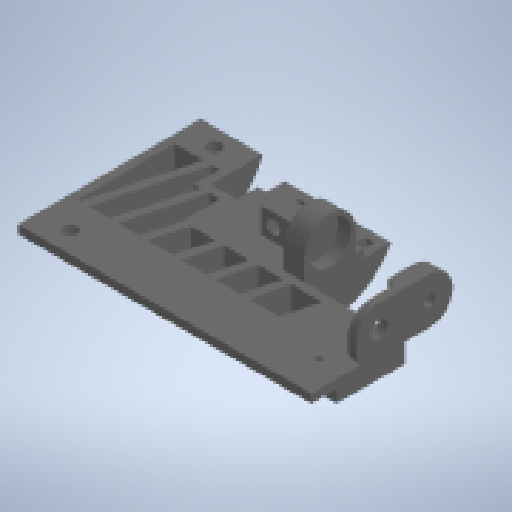
# Autodesk Inventor part: hand_motor_setter_cover_under
Saved by Autodesk Inventor 2024.1 (Build 281209000, 209)
## iProperties
Created: 2025-01-23
Part Number: hand_motor_setter_cover_under
Material: 一般
Document SubType Name: Modeling
Designer: hibik
Density: 1 g/cm^3
Appearance: 既定
Author: hibik
Autodesk Inventor part; units mm, degrees
ref_plane "YZ Plane" through (0, 0, 0) normal (1, 0, 0) x (0, 1, 0)
ref_plane "XZ Plane" through (0, 0, 0) normal (0, 1, 0) x (-1, 0, 0)
sketch "スケッチ1" plane through (0, 0, 0) normal (0, 1, 0) x (-1, 0, 0)
  line L0 (0, 0) -> (-14.7, 0)
  line L1 (-14.7, 0) -> (-14.7, -44.2)
  line L2 (-14.7, -44.2) -> (0, -44.2)
  line L3 (0, -44.2) -> (0, 0)
  line L4 (-14.7, -36.2) -> (-69.7, -36.2)
  line L5 (-69.7, -36.2) -> (-69.7, -22.1)
  line L6 (-69.7, -22.1) -> (-14.7, -22.1)
  line L7 (-14.7, -22.1) -> (-14.7, -36.2)
  line L8 (-7.35, -44.2) -> (-7.35, 0) construction
  circle A0 centre (-7.35, -39.2) radius 1.6
  circle A1 centre (-7.35, -5) radius 1.6
  point P0 (-14.7, -22.1)
  dimension "d0" = 14.7
  dimension "d1" = 44.2
  dimension "d2" = 22.1
  dimension "d3" = 14.1
  dimension "d4" = 3.2
  dimension "d5" = 3.2
  dimension "d6" = 5
  dimension "d7" = 5
  dimension "d20" = 55
  constraints: 18 end point, 4 parallel, 3 point on line, 2 centre point, 2 horizontal, 2 midpoint, 2 perpendicular
  measures "d0" distance of L2.end L1.end
  measures "d1" distance of L1.end L0.end
  measures "d2" distance between parallel lines of L2 L6
  measures "d3" distance between parallel lines of L6 L4
  measures "d4" diameter of A0
  measures "d5" diameter of A1
  measures "d6" distance of L8.start A0.centre
  measures "d7" distance from line of L0 A1.centre
  measures "d20" distance of L4.start L4.end
extrude "押し出し1" add sketch "スケッチ1" along normal blind 2
ref_plane "作業平面1" through (31, 0, -44.2) normal (-1, 0, 0) x (0, 0, 1)
sketch "スケッチ3" plane through (31, 0, -44.2) normal (-1, 0, 0) x (0, 0, 1)
  line L0 (22.1, 0) -> (8, 0) projected
  line L1 (8, 0) -> (8, 2) projected
  line L2 (22.1, 2) -> (8, 2) projected
  line L3 (22.1, 0) -> (22.1, 2) projected
  line L4 (17.45, 2) -> (12.65, 2)
  line L5 (12.65, 2) -> (12.65, 8)
  line L6 (12.65, 8) -> (17.45, 8)
  line L7 (17.45, 8) -> (17.45, 2)
  line L8 (22.1, 0) -> (8, 0) projected
  point P0 (44.2, 0)
  point P1 (15.05, 8)
  point P2 (15.05, 0)
  point P3 (12.65, 2)
  dimension "d11" = 4.8
  dimension "d12" = 6
  constraints: 8 end point, 2 midpoint, 2 parallel, 1 horizontal, 1 perpendicular, 1 point on line, 1 vertical alignment
  measures "d11" distance of L5.end L6.end
  measures "d12" distance of L6.end L4.start
extrude "押し出し2" add sketch "スケッチ3" against normal blind 5.9 contours L2 L5 L6 L7
sketch "スケッチ4" plane through (31, 2, -26.75) normal (0, 0, 1) x (1, 0, 0)
  circle A0 centre (2.9, 3) radius 1.6
  line L0 (5.9, 6) -> (5.9, 0) projected
  line L1 (0, 6) -> (5.9, 6) projected
  point P0 (-31, -2)
  dimension "d15" = 3.2
  dimension "d16" = 3
  dimension "d17" = 3
  constraints: 1 centre point
  measures "d15" diameter of A0
  measures "d16" distance from line of L0 A0.centre
  measures "d17" distance from line of L1 A0.centre
extrude "押し出し3" cut sketch "スケッチ4" against normal through all
sketch "スケッチ5" plane through (69.7, 0, -22.1) normal (1, 0, 0) x (0, 0, -1)
  circle A0 centre (-6, 7.1) radius 2 projected
  line L0 (0, 0) -> (14.1, 0) projected
  line L1 (14.1, 0) -> (14.1, 2) projected
  line L2 (0, 2) -> (14.1, 2) projected
  line L3 (0, 0) -> (0, 2) projected
  line L4 (14.1, 0) -> (22.1, 0) projected
  line L5 (14.1, 0) -> (-11.5, 0)
  line L6 (-11.5, 0) -> (-11.5, 12.6)
  line L7 (-11.5, 12.6) -> (14.1, 12.6)
  line L8 (14.1, 12.6) -> (14.1, 0)
  circle A1 centre (-6, 7.1) radius 5.5
  circle A2 centre (-6, 5.5) radius 5.5
  point P0 (-22.1, 0)
  point P1 (-11.5, 7.1)
  point P2 (-6, 12.6)
  point P3 (-11.5, 5.5)
  point P4 (-6, 0)
  dimension "d21" = 5.5
  dimension "d22" = 5.5
  constraints: 8 end point, 3 tangent, 2 centre point, 2 parallel, 1 coincident, 1 equal radius, 1 horizontal, 1 perpendicular
  measures "d21" distance from line of L6 A0.centre
  measures "d22" distance from line of L7 A0.centre
extrude "押し出し4" add sketch "スケッチ5" against normal blind 2 contours L3 L2 L1 L0 | L5 A2 A1 L7 L8 L2 L3 | A2 A1 | L6 A1 A2 | A1 A2 | A2 A1
sketch "スケッチ6" plane through (0, 0, 0) normal (0, -1, 0) x (1, 0, 0)
  line L0 (14.7, 0) -> (69.7, 0)
  line L1 (69.7, 0) -> (69.7, -22.1)
  line L2 (69.7, -22.1) -> (14.7, -22.1)
  line L3 (14.7, -22.1) -> (14.7, 0)
  line L4 (14.7, -22.1) -> (67.7, -22.1) projected
  line L5 (69.7, -16.1) -> (69.7, -36.2) projected
  point P0 (0, 0)
  constraints: 8 end point, 2 parallel, 1 coincident, 1 collinear, 1 horizontal, 1 perpendicular, 1 point on line
extrude "押し出し5" add sketch "スケッチ6" against normal up to surface (2 mm away)
sketch "スケッチ7" plane through (31, 2, -31.55) normal (0, 0, -1) x (-1, 0, 0)
  line L0 (-5.9, 0) -> (-5.9, 6) projected
  line L1 (-5.9, 6) -> (-36.7, 6)
  line L2 (-36.7, 6) -> (-36.7, 0)
  line L3 (-36.7, 0) -> (-5.9, 0)
  line L4 (-5.9, 0) -> (-5.9, 6)
  line L5 (-36.7, 10.6) -> (-36.7, 0) projected
  line L6 (-36.7, 0) -> (16.3, 0) projected
  point P0 (31, -2)
  point P1 (-36.7, 3)
  point P2 (-33.7, 0)
  constraints: 8 end point, 2 collinear, 2 parallel, 1 horizontal, 1 perpendicular
extrude "押し出し6" add sketch "スケッチ7" against normal up to surface (4.8 mm away)
ref_plane "作業平面2" through (41, 0, -44.2) normal (-1, 0, 0) x (0, 0, 1)
sketch "スケッチ8" plane through (41, 0, -44.2) normal (-1, 0, 0) x (0, 0, 1)
  circle A0 centre (16.1, 7.1) radius 2
  circle A1 centre (16.1, 7.1) radius 6
  line L0 (0, 2) -> (44.2, 2) projected
  line L1 (22.1, 7.1) -> (22.1, 2)
  line L2 (10.1, 7.1) -> (10.1, 0.8912)
  point P0 (44.2, 0)
  point P1 (10.1, 2)
  dimension "d38" = 12
  constraints: 4 end point, 2 centre point, 2 perpendicular, 2 point on circle, 2 tangent, 1 coincident, 1 midpoint, 2 other
  measures "d38" diameter of A1
extrude "押し出し7" add sketch "スケッチ8" against normal blind 5 contours A0 | A1 L0 | L1 L0 A1 | A1 L0 L2 picked at (16.1804, 3.0382)
sketch "スケッチ9" plane through (46, 0, -44.2) normal (1, 0, 0) x (0, 0, -1)
  line L0 (-12.65, 8) -> (-17.45, 8) projected
  line L1 (-12.65, 2) -> (-12.65, 8) projected
  line L2 (-17.45, 8) -> (-17.45, 2) projected
  line L3 (-12.55, 2) -> (-17.55, 2)
  point P0 (-44.2, 0)
  constraints: 2 end point, 1 horizontal, 2 other
extrude "押し出し8" cut sketch "スケッチ9" along normal blind 15
sketch "スケッチ10" plane through (0, 2, 0) normal (0, 1, 0) x (1, 0, 0)
  line L0 (46, 22.1) -> (46, 34.1) projected
  line L1 (46, 22.1) -> (61, 22.1)
  line L2 (61, 22.1) -> (61, 36.2)
  line L3 (61, 36.2) -> (46, 36.2)
  line L4 (46, 36.2) -> (46, 22.1)
  line L5 (61, 31.55) -> (61, 26.75) projected
  line L6 (67.7, 36.2) -> (14.7, 36.2) projected
  line L7 (19.8, 34.2) -> (14.8, 34.2)
  line L8 (14.7, 36.2) -> (19.8, 36.2)
  line L9 (19.8, 36.2) -> (19.8, 34.2)
  line L10 (19.8, 34.2) -> (14.7, 34.2)
  line L11 (14.7, 34.2) -> (14.7, 36.2)
  line L12 (19.8, 34.2) -> (20.8, 34.2)
  line L13 (20.8, 34.2) -> (20.8, 36.2)
  line L14 (20.8, 36.2) -> (19.8, 36.2)
  line L15 (19.8, 36.2) -> (19.8, 34.2)
  point P0 (0, 0)
  point P1 (64.7, 36.2)
  dimension "d37" = 1
  constraints: 26 end point, 6 parallel, 4 horizontal, 3 perpendicular, 2 collinear, 1 point on line, 2 other
  measures "d37" distance between parallel lines of L9 L13
extrude "押し出し9" cut sketch "スケッチ10" against normal through all
sketch "スケッチ11" plane through (46, 0, -44.2) normal (1, 0, 0) x (0, 0, -1)
  arc A0 (-10.1, 7.1) -> (-22.1, 7.1) centre (-16.1, 7.1) ccw projected
  circle A1 centre (-16.1, 7.1) radius 5
  point P0 (-44.2, 0)
  dimension "d39" = 10
  constraints: 1 centre point, 1 coincident
  measures "d39" diameter of A1
extrude "押し出し10" cut sketch "スケッチ11" against normal blind 3
sketch "スケッチ12" plane through (67.7, 0, -22.1) normal (-1, 0, 0) x (0, 0, 1)
  line L0 (0, 2) -> (0, 7.1) projected
  line L1 (6, 12.6) -> (-14.1, 12.6) projected
  line L2 (0, 2) -> (-14.1, 2)
  line L3 (-14.1, 2) -> (-14.1, 12.6)
  line L4 (-14.1, 12.6) -> (0, 12.6)
  line L5 (0, 12.6) -> (0, 2)
  point P0 (22.1, 0)
  point P1 (0, 7.1)
  constraints: 8 end point, 2 parallel, 1 horizontal, 1 perpendicular
extrude "押し出し11" add sketch "スケッチ12" along normal blind 3
fillet "フィレット3" radius 2.5 6 edges at (64.7, 2, -24.425) (62.85, 2, -26.75) (62.85, 8, -26.75) (62.85, 8, -31.55) (62.85, 2, -31.55) (64.7, 2, -33.875)
sketch "スケッチ13" plane through (61, 0, -44.2) normal (-1, 0, 0) x (0, 0, 1)
  circle A0 centre (15.05, 5.504) radius 1.6
  circle A1 centre (15.05, 5.504) radius 1.35
  point P0 (44.2, 0)
  dimension "d46" = 2.7
  constraints: 2 centre point, 1 coincident, 2 other
  measures "d46" diameter of A1
extrude "押し出し12" cut sketch "スケッチ13" against normal through all contours A1
sketch "スケッチ14" plane through (0, 0, 0) normal (0, -1, 0) x (1, 0, 0)
  circle A0 centre (63.3, -17.5) radius 1.25
  line L0 (69.7, 0) -> (69.7, -36.2) projected
  line L1 (54.7, -22.1) -> (69.7, -22.1)
  line L2 (69.7, -22.1) -> (69.7, -6)
  line L3 (69.7, -6) -> (54.7, -6)
  line L4 (54.7, -6) -> (54.7, -22.1)
  line L5 (46, -22.1) -> (61, -22.1) projected
  circle A1 centre (63.3, -8) radius 1.25
  circle A2 centre (63.3, -8) radius 0.85
  circle A3 centre (63.3, -17.5) radius 0.85
  point P0 (0, 0)
  dimension "d49" = 15
  dimension "d50" = 2
  dimension "d53" = 1.7
  dimension "d54" = 1.7
  constraints: 8 end point, 4 centre point, 2 coincident, 2 parallel, 1 collinear, 1 horizontal, 1 perpendicular, 1 point on line, 4 other
  measures "d49" distance of L1.start L1.end
  measures "d50" distance from line of L3 A1.centre
  measures "d53" diameter of A2
  measures "d54" diameter of A3
extrude "押し出し13" add sketch "スケッチ14" along normal blind 3 contours A0 | L0 L1 L4 L3 | A1
sketch "スケッチ15" plane through (0, -3, 0) normal (0, -1, 0) x (1, 0, 0)
  circle A0 centre (63.3, -8) radius 0.85 projected
  circle A1 centre (63.3, -17.5) radius 0.85 projected
  point P0 (0, 0)
extrude "押し出し14" cut sketch "スケッチ15" against normal through all
sketch "スケッチ16" plane through (0, 0, 0) normal (0, -1, 0) x (1, 0, 0)
  line L0 (50.9112, -3.9192) -> (55.6, -21.675)
  line L1 (51.5091, -10.1) -> (54.678, -22.1)
  line L2 (61, -22.1) -> (46, -22.1) projected
  line L3 (52.5434, -10.1) -> (46, -10.1)
  line L4 (46, -10.1) -> (46, -22.1)
  point P0 (0, 0)
  dimension "d57" = 1
  dimension "d58" = 12
  constraints: 8 end point, 3 point on line, 1 horizontal, 1 parallel, 1 perpendicular, 3 other
  measures "d57" distance between parallel lines of L0 L1
  measures "d58" distance between parallel lines of L2 L3
extrude "押し出し15" add sketch "スケッチ16" along normal blind 10
sketch "スケッチ17" plane through (0, 0, -44.2) normal (-1, 0, 0) x (0, 0, 1)
  arc A0 (12.7165, 22.8) -> (0.8318, 2) centre (16.05, 7.1) ccw
  circle A1 centre (16.05, 7.1) radius 16.05
  line L0 (16.05, -8.95) -> (34.1, -8.95)
  line L1 (34.1, 0) -> (34.1, -10) projected
  line L2 (0, 0) -> (44.2, 0) projected
  point P0 (1.6558, 0)
  constraints: 2 end point, 2 horizontal, 2 point on circle, 1 centre point, 1 point on line, 9 other
extrude "押し出し16" add sketch "スケッチ17" against normal up to surface (46 mm away) contours L2 A1 | L2 L1 L0 A1
sketch "スケッチ18" plane through (0, 0, 0) normal (-1, 0, 0) x (0, 0, 1)
  line L0 (-44.2, 0) -> (-42.5442, 0) projected
  arc A0 (-43.3682, 2) -> (-42.5442, 0) centre (-28.15, 7.1) ccw
  arc A1 (-42.5442, 0) -> (-28.15, -8.95) centre (-28.15, 7.1) ccw projected
  line L1 (-44.2, 2) -> (0, 2) projected
  line L2 (-44.2, 0) -> (-44.2, 2) projected
  point P0 (0, 0)
  constraints: 2 concentric, 2 point on circle, 1 centre point, 1 point on line
extrude "押し出し17" cut sketch "スケッチ18" against normal through all
sketch "スケッチ19" plane through (46, -10, -22.1) normal (-1, 0, 0) x (0, 0, 1)
  line L0 (12, 1.05) -> (0, 1.05) projected
  line L1 (0, 1.05) -> (0, 0) projected
  line L2 (12, 0) -> (0, 0) projected
  line L3 (12, 1.05) -> (12, 0) projected
  point P0 (22.1, 10)
extrude "押し出し18" cut sketch "スケッチ19" against normal through all
sketch "スケッチ20" plane through (0, -3, 0) normal (0, -1, 0) x (1, 0, 0)
  line L0 (0, -10.1) -> (51.5091, -10.1) projected
  line L1 (51.5091, -10.1) -> (54.7, -10.1)
  line L2 (54.7, -6) -> (54.7, -22.1) projected
  line L3 (51.5091, -10.1) -> (54.678, -22.1) projected
  line L4 (51.5091, -10.1) -> (54.678, -22.1)
  line L5 (54.7, -22.1) -> (69.7, -22.1) projected
  line L6 (69.7, -22.1) -> (69.7, -6) projected
  line L7 (69.7, -6) -> (54.7, -6) projected
  line L8 (54.7, -6) -> (54.7, -22.1) projected
  circle A0 centre (63.3, -17.5) radius 0.85 projected
  circle A1 centre (63.3, -8) radius 0.85 projected
  line L9 (54.678, -22.1) -> (54.7, -22.1)
  line L10 (61, -22.1) -> (46, -22.1) projected
  point P0 (0, 0)
  constraints: 6 end point, 2 collinear, 1 horizontal, 1 point on line
extrude "押し出し19" add sketch "スケッチ20" against normal up to surface (3 mm away)
sketch "スケッチ21" plane through (20.8, 0, -36.2) normal (0, 1, 0) x (1, 0, 0)
  line L0 (-6.1, 6.3442) -> (-6.1, -2) projected
  line L1 (-6.1, -2) -> (0, -2) projected
  line L2 (0, -2) -> (0, 0) projected
  line L3 (25.2, 0) -> (0, 0) projected
  line L4 (25.2, 6.3442) -> (25.2, 0) projected
  line L5 (-6.1, 6.3442) -> (25.2, 6.3442) projected
  line L6 (0, 0) -> (0, 6.3442)
  point P0 (-20.8, -36.2)
  constraints: 2 end point, 1 perpendicular, 1 point on line
extrude "押し出し20" cut sketch "スケッチ21" against normal through all contours L5 L6 L2 L1 L0
sketch "スケッチ22" plane through (20.8, 2, -34.2) normal (0, 0, -1) x (-1, 0, 0)
  line L0 (6.1, 0) -> (6.1, -9.7661) projected
  line L1 (0, 0) -> (6.1, 0) projected
  line L2 (0, 0) -> (0, -9.7661) projected
  line L3 (6.1, -9.7661) -> (0, -9.7661) projected
  line L4 (6.1, -9.7661) -> (0, -9.7661)
  line L5 (0, -9.7661) -> (0, -39.6948)
  line L6 (0, -39.6948) -> (6.1, -39.6948)
  line L7 (6.1, -39.6948) -> (6.1, -9.7661)
  line L8 (0, 0) -> (0, -9.7661) projected
  point P0 (20.8, -2)
  constraints: 8 end point, 2 parallel, 1 collinear, 1 horizontal, 1 perpendicular
extrude "押し出し21" cut sketch "スケッチ22" against normal blind 3
sketch "スケッチ23" plane through (0, 0, 0) normal (0, -1, 0) x (1, 0, 0)
  circle A0 centre (7.35, -39.2) radius 1.6 projected
  circle A1 centre (7.35, -39.2) radius 3
  point P0 (0, 0)
  dimension "d76" = 6
  constraints: 1 centre point, 1 coincident
  measures "d76" diameter of A1
extrude "押し出し22" cut sketch "スケッチ23" along normal through all contours A0 | A1
sketch "スケッチ24" plane through (0, 2, 0) normal (0, 1, 0) x (1, 0, 0)
  circle A0 centre (7.35, 5) radius 1.6 projected
  circle A1 centre (7.35, 39.2) radius 1.6 projected
  circle A2 centre (63.3, 17.5) radius 0.85 projected
  circle A3 centre (63.3, 8) radius 0.85 projected
  line L0 (20.8, 36.2) -> (20.8, 31.2) projected
  line L1 (20.8, 31.2) -> (14.7, 31.2) projected
  line L2 (14.7, 31.2) -> (14.7, 43.3682) projected
  line L3 (14.7, 43.3682) -> (0, 43.3682) projected
  line L4 (0, 43.3682) -> (0, 0) projected
  line L5 (0, 0) -> (69.7, 0) projected
  line L6 (69.7, 11.8574) -> (69.7, 0) projected
  line L7 (67.7, 11.8574) -> (69.7, 11.8574) projected
  line L8 (67.7, 22.1) -> (67.7, 11.8574) projected
  line L9 (67.7, 22.1) -> (62.2, 22.1) projected
  line L10 (62.2, 24.25) -> (62.2, 22.1) projected
  line L11 (61, 24.25) -> (62.2, 24.25) projected
  line L12 (61, 24.25) -> (61, 22.1) projected
  line L13 (61, 22.1) -> (46, 22.1) projected
  line L14 (46, 22.1) -> (41, 22.1) projected
  line L15 (41, 22.1) -> (41, 26.75) projected
  line L16 (41, 26.75) -> (31, 26.75) projected
  line L17 (31, 26.75) -> (31, 31.55) projected
  line L18 (31, 31.55) -> (41, 31.55) projected
  line L19 (41, 31.55) -> (41, 34.1) projected
  line L20 (41, 34.1) -> (46, 34.1) projected
  line L21 (46, 34.1) -> (46, 36.2) projected
  line L22 (46, 36.2) -> (20.8, 36.2) projected
  line L23 (20.8, 42.5442) -> (20.8, 36.2) projected
  line L24 (46, 36.2) -> (20.8, 36.2) projected
  line L25 (46, 42.5442) -> (46, 36.2) projected
  line L26 (20.8, 42.5442) -> (46, 42.5442) projected
  line L27 (0, 10.1) -> (51.5091, 10.1) projected
  line L28 (54.7, 10.1) -> (51.5091, 10.1) projected
  line L29 (54.7, 6) -> (54.7, 10.1) projected
  line L30 (69.7, 6) -> (54.7, 6) projected
  line L31 (20.8, 36.2) -> (41, 36.2)
  line L32 (41, 36.2) -> (41, 22.1)
  line L33 (41, 22.1) -> (20.8, 22.1)
  line L34 (20.8, 22.1) -> (20.8, 36.2)
  line L35 (17.75, 31.2) -> (69.7, 31.2)
  line L36 (69.7, 20.1) -> (18.8, 20.1)
  line L37 (18.8, 20.1) -> (18.8, 31.2)
  line L38 (20.8, 31.2) -> (14.7, 31.2) projected
  circle A4 centre (7.35, 39.2) radius 4
  line L39 (2, 35.2) -> (12.7, 35.2)
  line L40 (12.7, 35.2) -> (12.7, 12.1)
  line L41 (12.7, 12.1) -> (2, 12.1)
  line L42 (2, 12.1) -> (2, 35.2)
  line L43 (18.8, 29.2) -> (12.7, 29.2)
  line L44 (12.7, 12.1) -> (49.9687, 12.1)
  line L45 (49.9687, 12.1) -> (52.0812, 20.1)
  line L46 (51.5091, 10.1) -> (54.678, 22.1) projected
  line L47 (18.8, 20.1) -> (16.6874, 12.1)
  line L48 (18.756, 12.1) -> (20.8686, 20.1)
  line L49 (26.756, 12.1) -> (28.8686, 20.1)
  line L50 (26.8, 20.1) -> (24.6874, 12.1)
  line L51 (34.756, 12.1) -> (36.8686, 20.1)
  line L52 (34.8, 20.1) -> (32.6874, 12.1)
  line L53 (42.756, 12.1) -> (44.8686, 20.1)
  line L54 (42.8, 20.1) -> (40.6874, 12.1)
  line L55 (11.8, 20.1) -> (9.6874, 12.1)
  line L56 (11.756, 12.1) -> (13.8686, 20.1)
  line L57 (5.7, 12.1) -> (42.9687, 12.1)
  line L58 (4.8, 20.1) -> (2.6874, 12.1)
  line L59 (4.756, 12.1) -> (6.8686, 20.1)
  line L60 (-1.3, 12.1) -> (35.9687, 12.1)
  line L61 (11.8, 20.1) -> (14.203, 29.2)
  line L62 (13.8686, 20.1) -> (16.2716, 29.2)
  line L63 (4.8, 20.1) -> (8.7875, 35.2)
  line L64 (6.7136, 19.513) -> (10.856, 35.2)
  dimension "d79" = 2
  dimension "d80" = 2
  dimension "d81" = 8
  dimension "d82" = 2
  dimension "d83" = 2
  dimension "d84" = 2
  dimension "d85" = 2
  dimension "d88" = 2
  dimension "d89" = 2
  dimension "d95" = 8
  dimension "d102" = 7
  constraints: 64 end point, 14 point on line, 9 parallel, 6 horizontal, 4 collinear, 3 perpendicular, 1 centre point, 1 coincident, 1 midpoint, 1 tangent, 35 other
  measures "d79" distance between parallel lines of L36 L33
  measures "d80" distance between parallel lines of L34 L37
  measures "d81" diameter of A4
  measures "d82" distance between parallel lines of L4 L42
  measures "d83" distance between parallel lines of L1 L43
  measures "d84" distance between parallel lines of L2 L40
  measures "d85" distance between parallel lines of L27 L41
  measures "d88" distance between parallel lines of L46 L45
  measures "d89" distance between parallel lines of L48 L47
  measures "d95" distance of L48.start L49.start
  measures "d102" distance of L36.end L55.start
extrude "押し出し23" cut sketch "スケッチ24" against normal through all contours L37 L47 L44 L40 L56 L62 L43 | L36 L50 L44 L48 | L61 L40 L43 | L41 L56 L40 | L40 L61 L55 L41 L59 L64 L39 | L36 L52 L44 L49 | L45 L44 L53 L36 | L42 L39 L63 L58 L41 | L36 L54 L44 L51
sketch "スケッチ25" plane through (0, -8.95, -28.15) normal (0, -1, 0) x (1, 0, 0)
  line L0 (20.8686, 8.05) -> (18.756, 16.05) projected
  line L1 (24.6874, 16.05) -> (26.8, 8.05) projected
  line L2 (28.8686, 8.05) -> (26.756, 16.05) projected
  line L3 (32.6874, 16.05) -> (34.8, 8.05) projected
  line L4 (36.8686, 8.05) -> (34.756, 16.05) projected
  line L5 (40.6874, 16.05) -> (42.8, 8.05) projected
  line L6 (20.8686, 8.05) -> (26.2673, -12.3942)
  line L7 (26.8, 8.05) -> (32.1987, -12.3942)
  line L8 (28.8686, 8.05) -> (34.8, 8.05) projected
  line L9 (28.8686, 8.05) -> (34.2673, -12.3942)
  line L10 (34.8, 8.05) -> (40.1987, -12.3942)
  line L11 (36.8686, 8.05) -> (42.2673, -12.3942)
  line L12 (22.8, 6.05) -> (44, 6.05)
  line L13 (44, 6.05) -> (44, -12.3942)
  line L14 (44, -12.3942) -> (22.8, -12.3942)
  line L15 (22.8, -12.3942) -> (22.8, 6.05)
  line L16 (46, 6.05) -> (46, 0) projected
  line L17 (20.8, -14.3942) -> (46, -14.3942) projected
  line L18 (20.8, -14.3942) -> (20.8, -3.05) projected
  line L19 (42.8, 8.05) -> (36.8686, 8.05) projected
  point P0 (0, 28.15)
  point P1 (37.3967, 6.05)
  point P2 (35.3281, 6.05)
  point P3 (29.3967, 6.05)
  point P4 (22.8, 0.7359)
  point P5 (27.3281, 6.05)
  dimension "d107" = 2
  dimension "d108" = 2
  dimension "d109" = 2
  dimension "d110" = 2
  constraints: 18 end point, 5 collinear, 5 point on line, 2 parallel, 1 horizontal, 1 perpendicular
  measures "d107" distance between parallel lines of L16 L13
  measures "d108" distance between parallel lines of L17 L14
  measures "d109" distance between parallel lines of L18 L15
  measures "d110" distance between parallel lines of L19 L12
extrude "押し出し24" cut sketch "スケッチ25" against normal up to surface (8.95 mm away) contours L15 L12 L7 L14 L6 | L9 L12 L10 L14 | L11 L12 L13 L14
sketch "スケッチ26" plane through (0, 0, 0) normal (0, -1, 0) x (1, 0, 0)
  line L0 (69.7, -22.1) -> (61, -22.1) projected
  line L1 (61, -22.1) -> (61, -36.2) projected
  line L2 (69.7, -36.2) -> (61, -36.2) projected
  line L3 (69.7, -22.1) -> (69.7, -36.2) projected
  point P0 (0, 0)
extrude "押し出し25" cut sketch "スケッチ26" against normal through all
sketch "スケッチ27" plane through (69.7, 0, 0) normal (1, 0, 0) x (0, 0, -1)
  circle A0 centre (28.1, 7.1) radius 3
  line L0 (22.1, 12.6) -> (33.6, 12.6)
  line L1 (33.6, 12.6) -> (33.6, 1.6)
  line L2 (33.6, 1.6) -> (22.1, 1.6)
  line L3 (22.1, 1.6) -> (22.1, 12.6)
  circle A1 centre (28.1, 7.1) radius 5.5
  line L4 (22.1, 12.6) -> (16.1, 12.6) projected
  line L5 (22.1, -3) -> (22.1, 12.6) projected
  circle A2 centre (28.1, 7.1) radius 1.35
  point P0 (0, 0)
  point P1 (28.1, 12.6)
  point P2 (28.1, 1.6)
  dimension "d115" = 2.7
  constraints: 8 end point, 3 centre point, 3 tangent, 2 coincident, 2 collinear, 2 parallel, 1 horizontal, 1 perpendicular, 2 other
  measures "d115" diameter of A2
extrude "押し出し26" add sketch "スケッチ27" against normal blind 4 contours A0 | L0 A1 L2 L3 | A1
fillet "フィレット4" radius 2 1 edges at (67.7, 7.3, -22.1)
equation "\"d22\" = d21"
equation "\"d80\" = d79"
equation "\"d82\" = d79"
equation "\"d83\" = d79"
equation "\"d84\" = d83"
equation "\"d85\" = d79"
equation "\"d88\" = d79"
equation "\"d89\" = d79"
equation "\"d108\" = d107"
equation "\"d109\" = d108"
equation "\"d110\" = d107"
